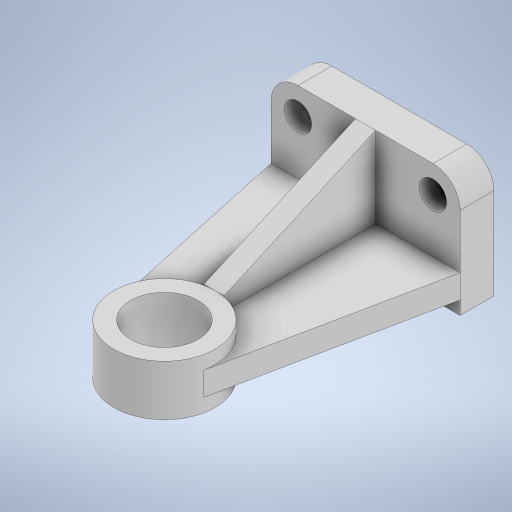
# Autodesk Inventor part: Soporte polea
Saved by Autodesk Inventor 2024 (Build 280153000, 153)
## iProperties
Created: 2024-03-03
Part Number: Soporte polea
Material: Genérico
Document SubType Name: Modeling
Designer: kelly
Density: 1 g/cm^3
Appearance: Valor por defecto
Author: kelly
Autodesk Inventor part; units mm, degrees
ref_plane "YZ Plane" through (0, 0, 0) normal (1, 0, 0) x (0, 1, 0)
ref_plane "XZ Plane" through (0, 0, 0) normal (0, 1, 0) x (-1, 0, 0)
sketch "Boceto1" plane through (0, 0, 0) normal (0, 0, 1) x (1, 0, 0)
  line L0 (-28, -17.5) -> (28, -17.5)
  line L1 (28, -17.5) -> (28, 9.5)
  line L2 (20, 17.5) -> (-20, 17.5)
  line L3 (-28, 9.5) -> (-28, -17.5)
  line L4 (-28, -17.5) -> (28, 17.5) construction
  line L5 (28, -17.5) -> (-28, 17.5) construction
  arc A0 (-20, 17.5) -> (-28, 9.5) centre (-20, 9.5) ccw
  arc A1 (28, 9.5) -> (20, 17.5) centre (20, 9.5) ccw
  circle A2 centre (-20, 9.5) radius 4
  circle A3 centre (20, 9.5) radius 4
  point P0 (0, 0)
  dimension "d0" = 56
  dimension "d1" = 35
  dimension "d2" = 8
  dimension "d3" = 8
  dimension "d4" = 8
  constraints: 12 end point, 4 centre point, 4 point on circle, 4 point on line, 4 tangent, 2 coincident, 2 midpoint, 2 parallel, 1 equal radius, 1 horizontal, 1 perpendicular
  measures "d0" distance of L5.end L4.end
  measures "d1" distance of L4.end L0.end
  measures "d2" radius of A0
  measures "d3" diameter of A2
  measures "d4" diameter of A3
extrude "Extrusión1" add sketch "Boceto1" along normal blind 10
ref_plane "Plano de trabajo2" through (-28, -13.5, 0) normal (0, -1, 0) x (1, 0, 0)
sketch "Boceto2" plane through (-28, -13.5, 0) normal (0, -1, 0) x (1, 0, 0)
  circle A0 centre (28.3324, 69.928) radius 15
  circle A1 centre (28.3324, 69.928) radius 10
  line L0 (8, 10) -> (0, 10) projected
  line L1 (0, 10) -> (13.6726, 73.1043)
  line L2 (56, 0) -> (56, 10) projected
  line L3 (56, 10) -> (43.0236, 72.9561)
  line L4 (0, 10) -> (56, 10)
  point P0 (28, 0)
  dimension "d8" = 30
  dimension "d9" = 20
  constraints: 6 end point, 2 centre point, 2 point on circle, 2 tangent, 1 coincident, 1 collinear
  measures "d8" diameter of A0
  measures "d9" diameter of A1
extrude "Extrusión2" add sketch "Boceto2" against normal blind 7 contours A0 L3 L4 L0 L1
extrude "Extrusión3" add sketch "Boceto2" against normal blind 11 contours A0
extrude "Extrusión4" add sketch "Boceto2" along normal blind 4 contours A0
sketch "Boceto3" plane through (0, 0, 0) normal (1, 0, 0) x (0, 1, 0)
  line L0 (9.5, 10) -> (-6.5, 10) projected
  line L1 (-6.5, 10) -> (17.5, 10)
  line L2 (17.5, 10) -> (-2.5, 54.928)
  line L3 (-17.5, 54.928) -> (-2.5, 54.928) projected
  line L4 (-6.5, 54.928) -> (-6.5, 10)
  line L5 (-6.5, 10) -> (-6.5, 73.1043) projected
  line L6 (-6.5, 54.928) -> (-2.5, 54.928)
  line L7 (-6.5, 54.928) -> (-6.5, 10)
  point P0 (0, 0)
  dimension "d17" = 24
  constraints: 10 end point, 3 collinear, 2 point on line, 1 perpendicular
  measures "d17" distance of L0.end L1.end
extrude "Extrusión5" add sketch "Boceto3" along normal mid plane 6
